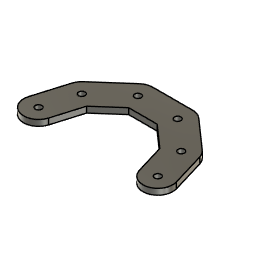
GearPlateV2 v6 (Autodesk Fusion 360 design; units mm, degrees)
Autodesk Fusion 360 part; units mm, degrees
sketch "Sketch1" plane through (0, 0, 0) normal (0, 0, 1) x (1, 0, 0)
  circle A0 centre (0, 0) radius 3.275
  circle A1 centre (120, 0) radius 3.275
  circle A2 centre (120, 0) radius 15 construction
  circle A3 centre (0, 0) radius 15 construction
  circle A4 centre (120, 0) radius 15 construction
  circle A5 centre (10, 33.541) radius 20 construction
  circle A6 centre (40, 59.9985) radius 20 construction
  circle A7 centre (110, 33.541) radius 20 construction
  circle A8 centre (80, 59.9985) radius 20 construction
  circle A9 centre (109.7709, 71.7327) radius 12 construction
  line L0 (143.6237, 88.934) -> (255.6237, 88.934) construction
  circle A10 centre (59.9233, -6.3144) radius 27.5 construction
  circle A11 centre (0, 0) radius 15 construction
  line L1 (150, 0) -> (-15, 0) construction
  circle A12 centre (0, 0) radius 17 construction
  circle A13 centre (120, 0) radius 17 construction
  circle A14 centre (10, 33.541) radius 3.275
  circle A15 centre (40, 59.9985) radius 3.275
  circle A16 centre (80, 59.9985) radius 3.275
  circle A17 centre (110, 33.541) radius 3.275
  circle A18 centre (0, 0) radius 15
  circle A19 centre (10, 33.541) radius 15
  circle A20 centre (40, 59.9985) radius 15
  circle A21 centre (80, 59.9985) radius 15
  circle A22 centre (110, 33.541) radius 15
  circle A23 centre (120, 0) radius 15
  line L2 (-14.3747, 4.2857) -> (-4.3747, 37.8267)
  line L3 (0.0784, 44.791) -> (30.0784, 71.2485)
  line L4 (40, 74.9985) -> (80, 74.9985)
  line L5 (14.3747, -4.2857) -> (24.3747, 29.2553)
  line L6 (19.9216, 22.291) -> (49.9216, 48.7485)
  line L7 (40, 44.9985) -> (80, 44.9985)
  line L8 (70.0784, 48.7485) -> (100.0784, 22.291)
  line L9 (89.9216, 71.2485) -> (119.9216, 44.791)
  line L10 (95.6253, 29.2553) -> (105.6253, -4.2857)
  line L11 (124.3747, 37.8267) -> (134.3747, 4.2857)
  point P0 (105, 0)
  point P1 (15, 0)
  dimension "d2" = 6.55
  dimension "d3" = 6.55
  dimension "d4" = 120
  dimension "d7" = 30
  dimension "d10" = 30
  dimension "d11" = 30
  dimension "d20" = 40
  dimension "d26" = 24
  dimension "d27" = 112
  dimension "d28" = 55
  dimension "d31" = 30
  dimension "d33" = 165
  dimension "d35" = 90
  dimension "d36" = 100
  dimension "d37" = 34
  dimension "d38" = 34
  dimension "d40" = 6.55
  dimension "d41" = 6.55
  dimension "d42" = 6.55
  dimension "d43" = 6.55
  dimension "d44" = 30
  dimension "d45" = 30
  dimension "d46" = 30
  dimension "d47" = 30
  dimension "d48" = 30
  dimension "d49" = 30
  constraint coincident A0.centre A3.centre
  constraint horizontal A0.centre A1.centre
  constraint concentric A1 A2
  constraint concentric A0 A3
  constraint concentric A1 A4
  constraint tangent A3 A5
  constraint tangent A4 A7
  constraint tangent A7 A8
  constraint tangent A6 A8
  constraint tangent A5 A6
  constraint tangent A8 A9
  constraint horizontal L0
  constraint horizontal A6.centre A8.centre
  constraint horizontal A5.centre A7.centre
  constraint concentric A3 A11
  constraint coincident A11 L1.end
  constraint horizontal L1
  constraint coincident A2 P0
  constraint coincident L1 P0
  constraint coincident A11 P1
  constraint coincident L1 P1
  constraint equal A5 A6
  constraint equal A6 A8
  constraint equal A7 A8
  constraint concentric A3 A12
  constraint concentric A4 A13
  constraint concentric A5 A14
  constraint concentric A6 A15
  constraint concentric A8 A16
  constraint concentric A7 A17
  constraint concentric A12 A18
  constraint concentric A14 A19
  constraint concentric A6 A20
  constraint concentric A16 A21
  constraint concentric A17 A22
  constraint concentric A1 A23
  constraint coincident A3 L2.start
  constraint coincident A19 L2.end
  constraint tangent A19 L2
  constraint coincident A19 L3.start
  constraint coincident A20 L3.end
  constraint tangent A20 L3
  constraint coincident A20 L4.start
  constraint coincident A21 L4.end
  constraint tangent A21 L4
  constraint coincident A3 L5.start
  constraint coincident A19 L5.end
  constraint tangent A19 L5
  constraint coincident A19 L6.start
  constraint coincident A20 L6.end
  constraint tangent A20 L6
  constraint coincident A20 L7.start
  constraint coincident A21 L7.end
  constraint tangent A21 L7
  constraint coincident A21 L8.start
  constraint coincident A22 L8.end
  constraint tangent A22 L8
  constraint coincident A21 L9.start
  constraint coincident A22 L9.end
  constraint tangent A22 L9
  constraint coincident A22 L10.start
  constraint coincident A2 L10.end
  constraint tangent A2 L10
  constraint coincident A22 L11.start
  constraint coincident A2 L11.end
  constraint tangent A2 L11
  constraint tangent A22 L11
  constraint tangent A22 L10
  constraint tangent A21 L8
  constraint tangent A21 L9
  constraint tangent A20 L4
  constraint tangent A20 L7
  constraint tangent A19 L6
  constraint tangent A3 L5
  constraint tangent A3 L2
  constraint tangent A19 L3
  measures "d2" diameter of A0
  measures "d3" diameter of A1
  measures "d4" distance of A0.centre A1.centre
  measures "d7" diameter of A2
  measures "d10" diameter of A3
  measures "d11" diameter of A4
  measures "d20" diameter of A5
  measures "d26" diameter of A9
  measures "d27" distance of L0.start L0.end
  measures "d28" diameter of A10
  measures "d31" diameter of A11
  measures "d33" distance of L1.start L1.end
  measures "d35" distance of P0 P1
  measures "d36" distance of A5.centre A7.centre
  measures "d37" diameter of A12
  measures "d38" diameter of A13
  measures "d40" diameter of A14
  measures "d41" diameter of A15
  measures "d42" diameter of A16
  measures "d43" diameter of A17
  measures "d44" diameter of A18
  measures "d45" diameter of A19
  measures "d46" diameter of A20
  measures "d47" diameter of A21
  measures "d48" diameter of A22
  measures "d49" diameter of A23
extrude "Extrude2" add sketch "Sketch1" along normal blind 6
equation "SlipGearNominal = 209.5 mm"
equation "d2 = HoleSize"
equation "d3 = HoleSize"
equation "SlipGearOffset = 0.5 mm"
equation "HoleSize = 6.55 mm"
equation "d40 = HoleSize"
equation "d41 = HoleSize"
equation "d42 = HoleSize"
equation "d43 = HoleSize"
